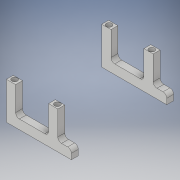
# Autodesk Inventor part: esp32_footprint_support
Saved by Autodesk Inventor 2019 (Build 230136000, 136)
## iProperties
Created: 2019-04-09
Part Number: esp32_footprint_support
Material: Generic
Document SubType Name: Modeling
Designer: jmc
Density: 1 g/cm^3
Appearance: Default
Author: jmc
## iProperties of the stored document esp32_footprint_3DPrint.ipt
Created: 2021-11-08
Part Number: esp32_footprint_3DPrint
Material: Genérico
Document SubType Name: Modeling
Designer: Juan M. Casillas
Density: 1 g/cm^3
Appearance: Valor por defecto
Author: Juan M. Casillas
Autodesk Inventor part; units mm, degrees
ref_plane "YZ Plane" through (0, 0, 0) normal (1, 0, 0) x (0, 1, 0)
ref_plane "XZ Plane" through (0, 0, 0) normal (0, 1, 0) x (-1, 0, 0)
ref_plane "XY Plane" through (0, 0, 0) normal (0, 0, 1) x (1, 0, 0)
sketch "Sketch1" plane through (0, 0, 0) normal (0, 1, 0) x (-1, 0, 0)
  line L0 (13.85, 27.5) -> (-13.85, 27.5)
  line L1 (-13.85, 27.5) -> (-13.85, -27.5)
  line L2 (-13.85, -27.5) -> (13.85, -27.5)
  line L3 (13.85, -27.5) -> (13.85, 27.5)
  line L4 (13.85, 27.5) -> (-13.85, -27.5) construction
  line L5 (-13.85, 27.5) -> (13.85, -27.5) construction
  line L6 (0, 27.5) -> (0, -27.5) construction
  line L7 (13.85, 0) -> (-13.85, 0) construction
  circle A0 centre (11.51, 25.4) radius 1.5
  circle A1 centre (11.51, -25.4) radius 1.5
  circle A2 centre (-11.51, 25.4) radius 1.5
  circle A3 centre (-11.51, -25.4) radius 1.5
  point P0 (0, 0)
  dimension "d0" = 27.7
  dimension "d1" = 55
  dimension "d2" = 3
  dimension "d3" = 2.34
  dimension "d4" = 2.1
  constraints: 16 end point, 6 midpoint, 4 centre point, 3 symmetric about line, 2 parallel, 1 horizontal, 1 perpendicular, 3 other
  measures "d0" distance of L2.end L1.end
  measures "d1" distance of L1.end L0.end
  measures "d2" diameter of A0
  measures "d3" distance from line of L3 A0.centre
  measures "d4" distance from line of L0 A0.centre
extrude "Extrusion1" add sketch "Sketch1" along normal blind 1
sketch "Sketch2" plane through (0, 1, 0) normal (0, 1, 0) x (1, 0, 0)
  circle A0 centre (11.51, 25.4) radius 1.5 projected
  circle A1 centre (11.51, -25.4) radius 1.5 projected
  circle A2 centre (-11.51, 25.4) radius 1.5 projected
  circle A3 centre (-11.51, -25.4) radius 1.5 projected
  line L0 (-13.85, -27.5) -> (13.85, -27.5) projected
  line L1 (13.85, -27.5) -> (13.85, 27.5) projected
  line L2 (13.85, 27.5) -> (-13.85, 27.5) projected
  line L3 (-13.85, 27.5) -> (-13.85, -27.5) projected
  point P0 (0, 0)
extrude "Extrusion2" add sketch "Sketch2" along normal blind 19
sketch "Sketch3" plane through (0, 20, 0) normal (0, 1, 0) x (1, 0, 0)
  line L0 (-13.85, 27.5) -> (-13.85, -27.5) projected
  line L1 (13.85, -27.5) -> (13.85, 27.5) projected
  line L2 (-13.85, -23.8) -> (13.85, -23.8)
  line L3 (13.85, -23.8) -> (13.85, 23.8)
  line L4 (13.85, 23.8) -> (-13.85, 23.8)
  line L5 (-13.85, 23.8) -> (-13.85, -23.8)
  line L6 (-13.85, -27.5) -> (13.85, -27.5) projected
  line L7 (13.85, 27.5) -> (-13.85, 27.5) projected
  point P0 (0, 0)
  dimension "d9" = 3.7
  dimension "d10" = 3.7
  constraints: 8 end point, 2 parallel, 2 point on line, 1 horizontal, 1 perpendicular
  measures "d9" distance between parallel lines of L6 L2
  measures "d10" distance between parallel lines of L7 L4
extrude "Extrusion3" cut sketch "Sketch3" against normal blind 20 contours L4 L1 L2 L0
sketch "Sketch4" plane through (-13.85, 0, 27.5) normal (0, 0, 1) x (1, 0, 0)
  line L0 (0, 0) -> (27.7, 0) projected
  line L1 (27.7, 20) -> (0, 20) projected
  line L2 (5, 0) -> (22.7, 0)
  line L3 (22.7, 0) -> (22.7, 20)
  line L4 (22.7, 20) -> (5, 20)
  line L5 (5, 20) -> (5, 0)
  line L6 (0, 0) -> (0, 20) projected
  line L7 (27.7, 0) -> (27.7, 20) projected
  point P0 (13.85, 0)
  dimension "d13" = 5
  dimension "d14" = 5
  constraints: 8 end point, 2 parallel, 2 point on line, 1 horizontal, 1 perpendicular
  measures "d13" distance between parallel lines of L6 L5
  measures "d14" distance between parallel lines of L7 L3
extrude "Extrusion4" cut sketch "Sketch4" against normal through all contours L5 L1 L3 L0
sketch "Sketch5" plane through (-8.85, 0, 27.5) normal (1, 0, 0) x (0, 0, -1)
  line L0 (3.7, 0) -> (0, 0) projected
  line L1 (3.7, 20) -> (3.7, 0) projected
  line L2 (0, 0) -> (3.7, 0)
  line L3 (3.7, 0) -> (3.7, 5)
  line L4 (3.7, 5) -> (0, 5)
  line L5 (0, 5) -> (0, 0)
  line L6 (51.3, 0) -> (51.3, 20) projected
  line L7 (55, 0) -> (55, 20) projected
  line L8 (51.3, 5) -> (55, 5)
  line L9 (55, 5) -> (55, 0)
  line L10 (55, 0) -> (51.3, 0)
  line L11 (51.3, 0) -> (51.3, 5)
  point P0 (27.5, 0)
  dimension "d17" = 5
  constraints: 16 end point, 4 parallel, 3 point on line, 2 horizontal, 2 perpendicular
  measures "d17" distance of L3.end L2.end
extrude "Extrusion5" add sketch "Sketch5" along normal blind 30
fillet "Fillet1" radius 2 8 edges at (-8.85, 5, 25.65) (13.85, 5, 25.65) (8.85, 5, 25.65) (21.15, 5, 25.65) (21.15, 5, -25.65) (13.85, 5, -25.65) (8.85, 5, -25.65) (-8.85, 5, -25.65)
equation "\"d10\" = d9"
equation "\"d14\" = d13"
body "Solid1"
